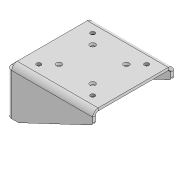
# Autodesk Inventor part: Plate_Angle
Saved by Autodesk Inventor 2020 (Build 240168000, 168)
## iProperties
Created: 2021-08-17
Part Number: Plate_Angle
Material: 一般
Document SubType Name: Sheet Metal
Designer: ken113
Density: 1 g/cm^3
Sheet Metal Rule: Default_mm
Appearance: 既定
Author: ken113
Autodesk Inventor part; units mm, degrees
ref_plane "YZ Plane" through (0, 0, 0) normal (1, 0, 0) x (0, 1, 0)
ref_plane "XZ Plane" through (0, 0, 0) normal (0, 1, 0) x (-1, 0, 0)
ref_plane "XY Plane" through (0, 0, 0) normal (0, 0, 1) x (1, 0, 0)
sketch "スケッチ1" plane through (0, 0, 0) normal (0, 1, 0) x (-1, 0, 0)
  line L0 (-30, 30) -> (30, 30)
  line L1 (30, 30) -> (30, -30)
  line L2 (30, -30) -> (-30, -30)
  line L3 (-30, -30) -> (-30, 30)
  line L4 (-30, 30) -> (30, -30) construction
  line L5 (30, 30) -> (-30, -30) construction
  point P0 (0, 0)
  dimension "d0" = 60
  dimension "d1" = 60
  measures "d0" distance of L0.start L0.end
  measures "d1" distance of L0.end L1.end
extrude "プレート1" add sketch "スケッチ1" along normal blind 2
sketch "スケッチ2" plane through (-30, 2, 28) normal (0, 0, 1) x (1, 0, 0)
  line L0 (60, 0) -> (0, 0)
  line L1 (0, 0) -> (0, -35)
  line L2 (0, -35) -> (60, -35)
  line L3 (60, -35) -> (60, 0)
  constraints: 6 end point, 1 horizontal, 1 perpendicular, 1 vertical
edge flange "フランジ1" height 35 angle 90 thickness 2 bend radius 2 thickness toward (0, 0, 1) relief tear relief width 2 relief depth 1 corner gap 2 corner form 0 edges at (0, 0, 30) (0, 0, -30) wall of the first edge with corners at (30, 2, 28) (-30, 2, 28) (-30, -33, 28) (30, -33, 28)
bend "曲げ1"
corner "コーナー1"
sketch "スケッチ3" plane through (-32, -2, 26) normal (-1, 0, 0) x (0, -1, 0)
  line L0 (31, 0) -> (0, 0)
  line L1 (0, 0) -> (0, -21)
  line L2 (0, -21) -> (31, -21)
  line L3 (31, -21) -> (31, 0)
  constraints: 6 end point, 1 horizontal, 1 perpendicular, 1 vertical
edge flange "フランジ2" height 25 angle 90 thickness 2 bend radius 2 thickness toward (-1, 0, 0) relief tear relief width 2 relief depth 1 corner gap 2 corner form 0 edges at (-30, -17.5, 28) (-30, -17.5, -28) wall of the first edge with corners at (-32, -33, 26) (-32, -2, 26) (-32, -2, 5) (-32, -33, 5)
bend "曲げ2"
corner "コーナー2"
sketch "スケッチ4" plane through (0, 2, 0) normal (0, 1, 0) x (1, 0, 0)
  line L0 (20, -20) -> (-20, -20)
  line L1 (-20, -20) -> (-20, 20)
  line L2 (-20, 20) -> (20, 20)
  line L3 (20, 20) -> (20, -20)
  line L4 (20, -20) -> (-20, 20) construction
  line L5 (-20, -20) -> (20, 20) construction
  point P0 (0, 0)
  dimension "d23" = 40
  dimension "d24" = 40
  constraints: 12 end point, 2 midpoint, 2 parallel, 1 horizontal, 1 perpendicular
  measures "d23" distance of L1.end L2.end
  measures "d24" distance of L0.end L1.end
hole "穴1" at (-20, 2, 20) at (20, 2, 20) at (20, 2, -20) at (-20, 2, -20) direction (0, -1, 0) diameter 3.242 end through all thread size "M4x0.7" class "6H" standard "ISO Metric profile"
sketch "スケッチ5" plane through (-32, -33, 5) normal (1, 0, 0) x (0, 0, -1)
  line L0 (-21, 31) -> (-21, 0) projected
  line L1 (0, 0) -> (-21, 0) projected
  line L2 (0, 0) -> (0, 31) projected
  line L3 (0, 31) -> (-21, 31) projected
  line L4 (31, 0) -> (31, 31) projected
  line L5 (10, 31) -> (31, 31) projected
  line L6 (10, 31) -> (10, 0) projected
  line L7 (10, 0) -> (31, 0) projected
  line L8 (-6, 6) -> (16, 6)
  line L9 (16, 6) -> (16, 25)
  line L10 (16, 25) -> (-6, 25)
  line L11 (-6, 25) -> (-6, 6)
  line L12 (-6, 6) -> (16, 25) construction
  line L13 (16, 6) -> (-6, 25) construction
  point P0 (5, 33)
  point P1 (5, 15.5)
  dimension "d32" = 6
  dimension "d33" = 6
  dimension "d34" = 6
  dimension "d35" = 6
  constraints: 12 end point, 2 midpoint, 2 parallel, 1 horizontal, 1 perpendicular
  measures "d32" distance between parallel lines of L2 L11
  measures "d33" distance between parallel lines of L9 L6
  measures "d34" distance between parallel lines of L8 L7
  measures "d35" distance between parallel lines of L5 L10
hole "穴2" at (-32, -8, 11) at (-32, -27, 11) at (-32, -27, -11) at (-32, -8, -11) direction (-1, 0, 0) diameter 5.2 end through all
fillet "フィレット1" radius 2 4 edges at (-33, -2, 5) (-33, -2, -5) (-33, -33, 5) (-33, -33, -5)
sketch "スケッチ6" plane through (30, -33, 30) normal (0, 0, 1) x (1, 0, 0)
  line L0 (0, 31) -> (-60, 31) projected
  line L1 (-60, 0) -> (-60, 31) projected
  line L2 (0, 0) -> (-60, 0) projected
  line L3 (0, 31) -> (0, 0) projected
  line L4 (-55, 0) -> (0, 26)
  point P0 (-30, 33)
  dimension "d44" = 5
  dimension "d45" = 5
  constraints: 2 end point, 2 point on line
  measures "d44" distance from line of L0 L4.end
  measures "d45" distance from line of L1 L4.start
extrude "押し出し1" cut sketch "スケッチ6" against normal through all contours L3 L2 L4
fillet "フィレット2" radius 2 4 edges at (-25, -33, 29) (-25, -33, -29) (30, -7, -29) (30, -7, 29)
sketch "スケッチ7" plane through (0, 2, 0) normal (0, 1, 0) x (1, 0, 0)
  line L0 (12.5, 12.5) -> (-12.5, 12.5)
  line L1 (-12.5, 12.5) -> (-12.5, -12.5)
  line L2 (-12.5, -12.5) -> (12.5, -12.5)
  line L3 (12.5, -12.5) -> (12.5, 12.5)
  line L4 (12.5, 12.5) -> (-12.5, -12.5) construction
  line L5 (-12.5, 12.5) -> (12.5, -12.5) construction
  point P0 (0, 0)
  dimension "d49" = 25
  dimension "d50" = 25
  constraints: 12 end point, 2 midpoint, 2 parallel, 1 horizontal, 1 perpendicular
  measures "d49" distance of L2.end L1.end
  measures "d50" distance of L1.end L0.end
hole "穴3" at (-12.5, 2, 12.5) at (12.5, 2, 12.5) at (12.5, 2, -12.5) at (-12.5, 2, -12.5) direction (0, -1, 0) diameter 4 end through all
equation "\"d56\" = Thickness"
equation "\"d2\" = Thickness"
equation "\"d3\" = BendReliefWidth"
equation "\"d4\" = BendReliefDepth"
equation "\"d5\" = MinimumRemnant"
equation "\"d6\" = TransitionRadius"
equation "\"d9\" = BendRadius"
equation "\"d10\" = CornerReliefSize"
equation "\"d11\" = GapSize"
equation "\"d12\" = JacobiRadiusSize"
equation "\"d13\" = BendReliefWidth"
equation "\"d14\" = BendReliefDepth"
equation "\"d15\" = MinimumRemnant"
equation "\"d16\" = TransitionRadius"
equation "\"d19\" = BendRadius"
equation "\"d20\" = CornerReliefSize"
equation "\"d21\" = GapSize"
equation "\"d22\" = JacobiRadiusSize"
equation "\"BendRadius\" = Thickness"
equation "\"BendReliefWidth\" = Thickness"
equation "\"BendReliefDepth\" = 0.5 * Thickness"
equation "\"CornerReliefSize\" = 4 * Thickness"
equation "\"MinimumRemnant\" = 2 * Thickness"
equation "\"TransitionRadius\" = BendRadius"
equation "\"JacobiRadiusSize\" = BendRadius"
equation "\"GapSize\" = Thickness"
equation "\"Thickness\" = 2"
